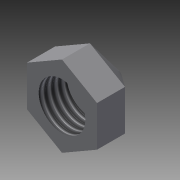
# Autodesk Inventor part: Nozzle
Saved by Autodesk Inventor 2014 SP1 (Build 180222100, 222)
## iProperties
Created: 2013-12-26
Part Number: Nozzle
Material: Generic
Document SubType Name: Modeling
Designer: Jack
Density: 1 g/cm^3
Appearance: Default
Author: Jack
Autodesk Inventor part; units mm, degrees
ref_plane "YZ Plane" through (0, 0, 0) normal (1, 0, 0) x (0, 1, 0)
ref_plane "XZ Plane" through (0, 0, 0) normal (0, 1, 0) x (-1, 0, 0)
sketch "Sketch1" plane through (0, 0, 0) normal (0, 1, 0) x (-1, 0, 0)
  line L0 (0, 8.6603) -> (7.5, 4.3301)
  line L1 (7.5, 4.3301) -> (7.5, -4.3301)
  line L2 (7.5, -4.3301) -> (0, -8.6603)
  line L3 (0, -8.6603) -> (-7.5, -4.3301)
  line L4 (-7.5, -4.3301) -> (-7.5, 4.3301)
  line L5 (-7.5, 4.3301) -> (0, 8.6603)
  point P0 (0, 0)
  point P1 (0, 0)
  dimension "d0" = 7.5
  constraints: 12 end point, 1 coincident, 1 vertical, 13 other
  measures "d0" distance from line of point (0, 0) L4
extrude "Extrusion1" add sketch "Sketch1" along normal blind 6
ref_plane "Work Plane1" through (0, 12, 0) normal (0, 1, 0) x (1, 0, 0)
sketch "Sketch3" plane through (0, 12, 0) normal (0, 1, 0) x (1, 0, 0)
  circle A0 centre (0, 0) radius 0.75
  dimension "d4" = 1.5
  constraints: 1 centre point, 1 coincident
  measures "d4" diameter of A0
loft "Loft1" add profiles "Sketch3" section 1 edges at (-3.75, 6, 6.4952) (3.75, 6, 6.4952) (7.5, 6, 0) (3.75, 6, -6.4952) (-3.75, 6, -6.4952) (-7.5, 6, 0)
sketch "Sketch4" plane through (0, 0, 0) normal (0, -1, 0) x (1, 0, 0)
  circle A0 centre (0, 0) radius 5
  dimension "d9" = 10
  constraints: 1 centre point, 1 coincident
  measures "d9" diameter of A0
extrude "Extrusion2" cut sketch "Sketch4" against normal blind 6
thread "Thread1" size "M10x1.5" class "6H" standard "ANSI Metric M Profile" full length
sketch "Sketch5" plane through (0, 6, 0) normal (0, -1, 0) x (1, 0, 0)
  circle A0 centre (0, 0) radius 5 projected
  circle A1 centre (0, 0) radius 1.5875
  dimension "d14" = 3.175
  constraints: 1 centre point, 1 coincident
  measures "d14" diameter of A1
sketch "Sketch6" plane through (0, 12, 0) normal (0, 1, 0) x (1, 0, 0)
  arc A0 (-0.6495, 0.375) -> (-0.6495, -0.375) centre (0, 0) ccw projected
  circle A1 centre (0, 0) radius 0.175
  dimension "d15" = 0.35
  constraints: 1 centre point, 1 coincident
  measures "d15" diameter of A1
extrude "Extrusion3" cut sketch "Sketch6" against normal blind 7.75
extrude "Extrusion4" cut sketch "Sketch5" against normal blind 3.9 contours A1
chamfer "Chamfer1" distance 1.4 angle 45 1 edges at (-0.175, 9.9, 0)
body "Solid1"
